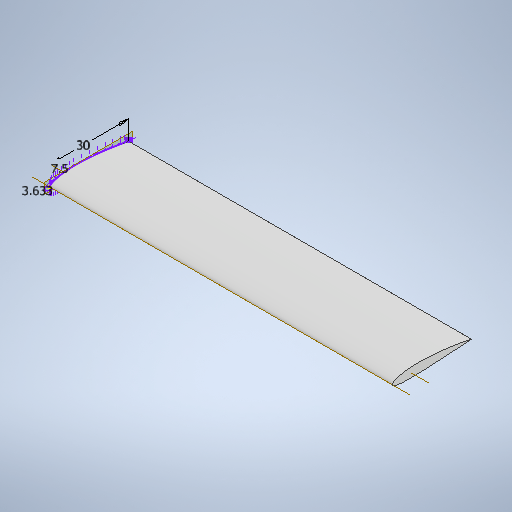
# Autodesk Inventor part: Wing
Saved by Autodesk Inventor 2027.1 (Build 311270010, 270A)
## iProperties
Created: 2026-09-09
Part Number: Wing
Material: Generic
Document SubType Name: Modeling
Designer: PWYNNE
Density: 1 g/cm^3
Appearance: Default
Author: PWYNNE
Autodesk Inventor part; units mm, degrees
ref_plane "YZ Plane" through (0, 0, 0) normal (1, 0, 0) x (0, 1, 0)
ref_plane "XZ Plane" through (0, 0, 0) normal (0, 1, 0) x (-1, 0, 0)
ref_plane "XY Plane" through (0, 0, 0) normal (0, 0, 1) x (1, 0, 0)
sketch "Sketch2" plane through (0, 0, 0) normal (1, 0, 0) x (0, 1, 0)
  spline S0 degree 4 poles (0.033, -299.9994) (3.3039, -286.0834) (4.2253, -281.644) (10.8718, -244.4612) (15.6087, -209.9801) (19.3174, -180.1453) (21.7757, -149.893) (23.6281, -124.1514) (23.8641, -91.2118) (23.2597, -77.4121) (21.9027, -60.0223) (20.308, -46.9169) (17.3008, -30.6814) (15.0451, -23.3554) (13.1157, -15.9301) (8.6543, -6.8941) (7.6022, -4.5563) (-0.1671, 2.9786) (-5.7327, -4.4664) (-6.7557, -7.0087) (-9.5953, -16.0457) (-10.5091, -23.3964) (-11.4863, -30.7759) (-12.5533, -47.0018) (-12.769, -60.0712) (-12.7192, -77.4452) (-12.3653, -91.2263) (-11.3734, -124.1322) (-10.1013, -149.8619) (-8.3197, -180.0808) (-6.4272, -209.9252) (-4.3358, -244.3423) (-1.5592, -281.5624) (-1.5901, -286.0631) (-0.033, -299.9994) knots 0 0 0 0 0 0.079222 0.116044 0.155717 0.19533 0.234892 0.271531 0.305271 0.336139 0.364181 0.390261 0.414415 0.436733 0.455834 0.474841 0.493268 0.510208 0.528357 0.546554 0.565216 0.587182 0.611089 0.637002 0.664944 0.695772 0.729497 0.766123 0.80565 0.845185 0.884726 0.921374 1 1 1 1 1
  line L0 (0.033, -299.9994) -> (-0.033, -299.9994)
  line L1 (-0.033, 0.0006) -> (0, -299.9994) construction
  line L2 (23.6234, -180.0002) -> (23.6234, 0.0006) construction
  line L3 (-12.7065, -120.0004) -> (-12.7065, 0.0006) construction
  point P0 (0, 0)
  point P1 (3.4035, -284.9994)
  point P2 (6.2235, -269.9995)
  point P3 (11.2335, -239.9995)
  point P4 (15.5235, -209.9996)
  point P5 (19.0635, -179.9996)
  point P6 (21.7034, -149.9997)
  point P7 (23.3834, -119.9998)
  point P8 (23.6234, -89.9998)
  point P9 (22.9934, -74.9998)
  point P10 (21.7634, -59.9999)
  point P11 (19.8134, -44.9999)
  point P12 (16.8735, -29.9999)
  point P13 (14.8635, -22.5)
  point P14 (12.3735, -15)
  point P15 (8.9535, -7.5)
  point P16 (6.4335, -3.75)
  point P17 (-4.9665, -3.75)
  point P18 (-6.8265, -7.5)
  point P19 (-9.0465, -15)
  point P20 (-10.3965, -22.5)
  point P21 (-11.2665, -29.9999)
  point P22 (-12.3165, -44.9999)
  point P23 (-12.7065, -59.9999)
  point P24 (-12.6765, -74.9998)
  point P25 (-12.3765, -89.9998)
  point P26 (-11.4165, -119.9998)
  point P27 (-10.0365, -149.9997)
  point P28 (-8.2965, -179.9996)
  point P29 (-6.4365, -209.9996)
  point P30 (-4.5165, -239.9995)
  point P31 (-2.4765, -269.9995)
  point P32 (-1.4565, -284.9994)
  point P33 (-0.0165, -149.9997)
  point P34 (-0.0165, -75)
  dimension "d0" = 75
  dimension "d1" = 300
  dimension "d2" = 36.3299
  constraints: 8 end point, 3 midpoint, 2 vertical, 37 other
  measures "d0" distance of point (0, 0) point (-0.017, -75)
  measures "d1" distance of L1.start L1.end
  measures "d2" distance between parallel lines of L3 L2
extrude "Extrusion1" add sketch "Sketch2" along normal blind 1300
ref_plane "Work Plane1" through (0, 0, 0) normal (-1, 0, 0) x (0, 0, 1)
ref_plane "Work Plane3" through (1300, 0.033, -74.9994) normal (0, 0, -1) x (-1, 0, 0)
ref_plane "Work Plane2" through (1300, 0.033, 0.0006) normal (0, 0, -1) x (-1, 0, 0)
body "Solid1"
